Autodesk Inventor part; units mm, degrees
(part 2 of 2)
  line L844 (361.7717, -1.1157) -> (362.4363, -1.1869)
  line L845 (362.4363, -1.1869) -> (363.102, -1.2506)
  line L846 (363.102, -1.2506) -> (363.7686, -1.3069)
  line L847 (363.7686, -1.3069) -> (364.4362, -1.3556)
  line L848 (364.4362, -1.3556) -> (365.1045, -1.3968)
  line L849 (365.1045, -1.3968) -> (365.7734, -1.4306)
  line L850 (365.7734, -1.4306) -> (366.4428, -1.4568)
  line L851 (366.4428, -1.4568) -> (367.1126, -1.4755)
  line L852 (367.1126, -1.4755) -> (367.7826, -1.4867)
  line L853 (367.7826, -1.4867) -> (368.4527, -1.4904)
  line L854 (368.4527, -1.4904) -> (369.1228, -1.4866)
  line L855 (369.1228, -1.4866) -> (369.7928, -1.4753)
  line L856 (369.7928, -1.4753) -> (370.4625, -1.4565)
  line L857 (370.4625, -1.4565) -> (371.1319, -1.4302)
  line L858 (371.1319, -1.4302) -> (371.8008, -1.3964)
  line L859 (371.8008, -1.3964) -> (372.469, -1.3551)
  line L860 (372.469, -1.3551) -> (373.1365, -1.3063)
  line L861 (373.1365, -1.3063) -> (373.8031, -1.25)
  line L862 (373.8031, -1.25) -> (374.4687, -1.1861)
  line L863 (374.4687, -1.1861) -> (375.1331, -1.1148)
  line L864 (375.1331, -1.1148) -> (375.7963, -1.036)
  line L865 (375.7963, -1.036) -> (376.4582, -0.9497)
  line L866 (376.4582, -0.9497) -> (377.1185, -0.8558)
  line L867 (377.1185, -0.8558) -> (377.7773, -0.7545)
  line L868 (377.7773, -0.7545) -> (378.4342, -0.6457)
  line L869 (378.4342, -0.6457) -> (379.0893, -0.5293)
  line L870 (379.0893, -0.5293) -> (379.7424, -0.4055)
  line L871 (379.7424, -0.4055) -> (380.3934, -0.2741)
  line L872 (380.3934, -0.2741) -> (381.0421, -0.1353)
  line L873 (381.0421, -0.1353) -> (381.6885, 0.0111)
  line L874 (381.6885, 0.0111) -> (382.3324, 0.1649)
  line L875 (382.3324, 0.1649) -> (382.9736, 0.3263)
  line L876 (382.9736, 0.3263) -> (383.6121, 0.4951)
  line L877 (383.6121, 0.4951) -> (384.2478, 0.6715)
  line L878 (384.2478, 0.6715) -> (384.8804, 0.8553)
  line L879 (384.8804, 0.8553) -> (385.5099, 1.0467)
  line L880 (385.5099, 1.0467) -> (386.1362, 1.2456)
  line L881 (386.1362, 1.2456) -> (386.7591, 1.4519)
  line L882 (386.7591, 1.4519) -> (387.3786, 1.6658)
  line L883 (387.3786, 1.6658) -> (387.9944, 1.8872)
  line L884 (387.9944, 1.8872) -> (388.6064, 2.116)
  line L885 (388.6064, 2.116) -> (389.2146, 2.3524)
  line L886 (389.2146, 2.3524) -> (414.1281, 2.3519)
  line L887 (414.1281, 2.3519) -> (414.4071, 2.3417)
  line L888 (414.4071, 2.3417) -> (414.6781, 2.3116)
  line L889 (414.6781, 2.3116) -> (414.9399, 2.2627)
  line L890 (414.9399, 2.2627) -> (415.191, 2.1959)
  line L891 (415.191, 2.1959) -> (415.4301, 2.1122)
  line L892 (415.4301, 2.1122) -> (415.6557, 2.0127)
  line L893 (415.6557, 2.0127) -> (415.8665, 1.8982)
  line L894 (415.8665, 1.8982) -> (416.061, 1.7698)
  line L895 (416.061, 1.7698) -> (416.2379, 1.6284)
  line L896 (416.2379, 1.6284) -> (416.3957, 1.4751)
  line L897 (416.3957, 1.4751) -> (416.5331, 1.3109)
  line L898 (416.5331, 1.3109) -> (416.6486, 1.1366)
  line L899 (416.6486, 1.1366) -> (416.741, 0.9533)
  line L900 (416.741, 0.9533) -> (416.8086, 0.7621)
  line L901 (416.8086, 0.7621) -> (416.8503, 0.5638)
  line L902 (416.8503, 0.5638) -> (416.8645, 0.3594)
  line L903 (416.8645, 0.3594) -> (416.8634, -6.4468)
  line L904 (416.8634, -6.4468) -> (416.5583, -7.6601)
  line L905 (416.5583, -7.6601) -> (416.263, -8.8753)
  line L906 (416.263, -8.8753) -> (415.9774, -10.0921)
  line L907 (415.9774, -10.0921) -> (415.7014, -11.3106)
  line L908 (415.7014, -11.3106) -> (415.4352, -12.5308)
  line L909 (415.4352, -12.5308) -> (415.1787, -13.7525)
  line L910 (415.1787, -13.7525) -> (414.932, -14.9757)
  line L911 (414.932, -14.9757) -> (414.6949, -16.2003)
  line L912 (414.6949, -16.2003) -> (414.4676, -17.4263)
  line L913 (414.4676, -17.4263) -> (414.2499, -18.6536)
  line L914 (414.2499, -18.6536) -> (414.042, -19.8822)
  line L915 (414.042, -19.8822) -> (413.8438, -21.1119)
  line L916 (413.8438, -21.1119) -> (413.6553, -22.3429)
  line L917 (413.6553, -22.3429) -> (413.4765, -23.5749)
  line L918 (413.4765, -23.5749) -> (413.3074, -24.8079)
  line L919 (413.3074, -24.8079) -> (413.1481, -26.042)
  line L920 (413.1481, -26.042) -> (412.9984, -27.2769)
  line L921 (412.9984, -27.2769) -> (412.8585, -28.5127)
  line L922 (412.8585, -28.5127) -> (412.7283, -29.7493)
  line L923 (412.7283, -29.7493) -> (412.6078, -30.9866)
  line L924 (412.6078, -30.9866) -> (412.497, -32.2247)
  line L925 (412.497, -32.2247) -> (412.3959, -33.4633)
  line L926 (412.3959, -33.4633) -> (412.3046, -34.7025)
  line L927 (412.3046, -34.7025) -> (412.2229, -35.9423)
  line L928 (412.2229, -35.9423) -> (412.151, -37.1824)
  line L929 (412.151, -37.1824) -> (412.0888, -38.423)
  line L930 (412.0888, -38.423) -> (412.0363, -39.6639)
  line L931 (412.0363, -39.6639) -> (411.9935, -40.9051)
  line L932 (411.9935, -40.9051) -> (411.9604, -42.1466)
  line L933 (411.9604, -42.1466) -> (411.937, -43.3882)
  line L934 (411.937, -43.3882) -> (411.9234, -44.6299)
  line L935 (411.9234, -44.6299) -> (411.9194, -45.8716)
  line L936 (411.9194, -45.8716) -> (411.9252, -47.1133)
  line L937 (411.9252, -47.1133) -> (411.9407, -48.355)
  line L938 (411.9407, -48.355) -> (411.9659, -49.5966)
  line L939 (411.9659, -49.5966) -> (412.0009, -50.8379)
  line L940 (412.0009, -50.8379) -> (412.0455, -52.079)
  line L941 (412.0455, -52.079) -> (412.0998, -53.3199)
  line L942 (412.0998, -53.3199) -> (412.1639, -54.5604)
  line L943 (412.1639, -54.5604) -> (412.2377, -55.8004)
  line L944 (412.2377, -55.8004) -> (412.3212, -57.04)
  line L945 (412.3212, -57.04) -> (412.4144, -58.2791)
  line L946 (412.4144, -58.2791) -> (412.5173, -59.5176)
  line L947 (412.5173, -59.5176) -> (412.63, -60.7554)
  line L948 (412.63, -60.7554) -> (412.7523, -61.9925)
  line L949 (412.7523, -61.9925) -> (412.8844, -63.2289)
  line L950 (412.8844, -63.2289) -> (413.0262, -64.4645)
  line L951 (413.0262, -64.4645) -> (413.1777, -65.6992)
  line L952 (413.1777, -65.6992) -> (413.3389, -66.9329)
  line L953 (413.3389, -66.9329) -> (413.5098, -68.1657)
  line L954 (413.5098, -68.1657) -> (413.6905, -69.3974)
  line L955 (413.6905, -69.3974) -> (413.8808, -70.628)
  line L956 (413.8808, -70.628) -> (414.0809, -71.8575)
  line L957 (414.0809, -71.8575) -> (414.2907, -73.0857)
  line L958 (414.2907, -73.0857) -> (414.5102, -74.3127)
  line L959 (414.5102, -74.3127) -> (414.7395, -75.5383)
  line L960 (414.7395, -75.5383) -> (414.9784, -76.7625)
  line L961 (414.9784, -76.7625) -> (415.227, -77.9853)
  line L962 (415.227, -77.9853) -> (415.4854, -79.2065)
  line L963 (415.4854, -79.2065) -> (415.7535, -80.4262)
  line L964 (415.7535, -80.4262) -> (416.0313, -81.6443)
  line L965 (416.0313, -81.6443) -> (416.3188, -82.8607)
  line L966 (416.3188, -82.8607) -> (416.616, -84.0753)
  line L967 (416.616, -84.0753) -> (416.923, -85.2882)
  line L968 (416.923, -85.2882) -> (416.8645, -89.6425)
  line L969 (416.8645, -89.6425) -> (416.8645, -95.6442)
  line L970 (416.8645, -95.6442) -> (416.8645, -105.6549)
  line L971 (416.8645, -105.6549) -> (416.8504, -105.8592)
  line L972 (416.8504, -105.8592) -> (416.8088, -106.0574)
  line L973 (416.8088, -106.0574) -> (416.7412, -106.2487)
  line L974 (416.7412, -106.2487) -> (416.649, -106.4319)
  line L975 (416.649, -106.4319) -> (416.5335, -106.6062)
  line L976 (416.5335, -106.6062) -> (416.3961, -106.7705)
  line L977 (416.3961, -106.7705) -> (416.2384, -106.9238)
  line L978 (416.2384, -106.9238) -> (416.0615, -107.0651)
  line L979 (416.0615, -107.0651) -> (415.867, -107.1936)
  line L980 (415.867, -107.1936) -> (415.6563, -107.3081)
  line L981 (415.6563, -107.3081) -> (415.4307, -107.4077)
  line L982 (415.4307, -107.4077) -> (415.1916, -107.4914)
  line L983 (415.1916, -107.4914) -> (414.9404, -107.5582)
  line L984 (414.9404, -107.5582) -> (414.6786, -107.6072)
  line L985 (414.6786, -107.6072) -> (414.4075, -107.6373)
  line L986 (414.4075, -107.6373) -> (414.1285, -107.6476)
  line L987 (414.1285, -107.6476) -> (322.7439, -107.6476)
  line L988 (322.7439, -107.6476) -> (322.4611, -107.6373)
  line L989 (322.4611, -107.6373) -> (322.1866, -107.6073)
  line L990 (322.1866, -107.6073) -> (321.9219, -107.5583)
  line L991 (321.9219, -107.5583) -> (321.6682, -107.4915)
  line L992 (321.6682, -107.4915) -> (321.427, -107.4078)
  line L993 (321.427, -107.4078) -> (321.1997, -107.3083)
  line L994 (321.1997, -107.3083) -> (320.9874, -107.1938)
  line L995 (320.9874, -107.1938) -> (320.7918, -107.0654)
  line L996 (320.7918, -107.0654) -> (320.614, -106.924)
  line L997 (320.614, -106.924) -> (320.4555, -106.7707)
  line L998 (320.4555, -106.7707) -> (320.3177, -106.6064)
  line L999 (320.3177, -106.6064) -> (320.2018, -106.4322)
  line L1000 (320.2018, -106.4322) -> (320.1093, -106.2489)
  line L1001 (320.1093, -106.2489) -> (320.0416, -106.0577)
  line L1002 (320.0416, -106.0577) -> (319.9999, -105.8594)
  line L1003 (319.9999, -105.8594) -> (319.9856, -105.655)
  line L1004 (319.9856, -105.655) -> (319.9856, -95.6442)
  line L1005 (0, 0) -> (1, 0)
  line L1006 (319.9856, -95.6442) -> (319.9856, -89.6425)
  line L1007 (319.9856, -89.6425) -> (319.9866, -88.8178)
  line L1008 (319.9866, -88.8178) -> (319.662, -88.8377)
  line L1009 (319.662, -88.8377) -> (319.3354, -88.8443)
  arc A21 (311.3354, -80.8443) -> (319.3354, -88.8443) centre (319.3354, -80.8443) ccw
  line L1010 (311.3354, -80.8443) -> (311.3452, -80.4456)
  line L1011 (311.3452, -80.4456) -> (311.3742, -80.052)
  line L1012 (311.3742, -80.052) -> (311.4219, -79.6638)
  line L1013 (311.4219, -79.6638) -> (311.488, -79.2816)
  line L1014 (311.488, -79.2816) -> (311.5719, -78.9059)
  line L1015 (311.5719, -78.9059) -> (311.6732, -78.537)
  line L1016 (311.6732, -78.537) -> (311.7915, -78.1755)
  line L1017 (311.7915, -78.1755) -> (311.9262, -77.8218)
  line L1018 (311.9262, -77.8218) -> (312.0769, -77.4763)
  line L1019 (312.0769, -77.4763) -> (312.2433, -77.1395)
  line L1020 (312.2433, -77.1395) -> (312.4247, -76.8119)
  line L1021 (312.4247, -76.8119) -> (312.6208, -76.494)
  line L1022 (312.6208, -76.494) -> (312.8311, -76.1861)
  line L1023 (312.8311, -76.1861) -> (313.0552, -75.8888)
  line L1024 (313.0552, -75.8888) -> (313.2926, -75.6024)
  line L1025 (313.2926, -75.6024) -> (313.5428, -75.3275)
  line L1026 (313.5428, -75.3275) -> (313.8053, -75.0646)
  line L1027 (313.8053, -75.0646) -> (314.0798, -74.814)
  line L1028 (314.0798, -74.814) -> (314.3658, -74.5762)
  line L1029 (314.3658, -74.5762) -> (314.6628, -74.3517)
  line L1030 (314.6628, -74.3517) -> (314.9703, -74.141)
  line L1031 (314.9703, -74.141) -> (315.2879, -73.9444)
  line L1032 (315.2879, -73.9444) -> (315.6152, -73.7625)
  line L1033 (315.6152, -73.7625) -> (315.9517, -73.5958)
  line L1034 (315.9517, -73.5958) -> (316.2968, -73.4446)
  line L1035 (316.2968, -73.4446) -> (316.6503, -73.3094)
  line L1036 (316.6503, -73.3094) -> (317.0116, -73.1907)
  line L1037 (317.0116, -73.1907) -> (317.3803, -73.089)
  line L1038 (317.3803, -73.089) -> (317.7558, -73.0047)
  line L1039 (317.7558, -73.0047) -> (318.1378, -72.9382)
  line L1040 (318.1378, -72.9382) -> (318.5258, -72.89)
  line L1041 (318.5258, -72.89) -> (318.9194, -72.8607)
  line L1042 (318.9194, -72.8607) -> (319.1155, -72.796)
  line L1043 (319.1155, -72.796) -> (319.2983, -72.7057)
  line L1044 (319.2983, -72.7057) -> (319.4657, -72.5919)
  line L1045 (319.4657, -72.5919) -> (319.6155, -72.4569)
  line L1046 (319.6155, -72.4569) -> (319.7458, -72.3027)
  line L1047 (319.7458, -72.3027) -> (319.8543, -72.1317)
  line L1048 (319.8543, -72.1317) -> (319.9389, -71.9458)
  line L1049 (319.9389, -71.9458) -> (319.9977, -71.7474)
  constraints: 2100 end point, 44 point on circle, 22 centre point, 1 coincident
extrude "Extrusión1" add sketch "Boceto1" along normal blind 5
